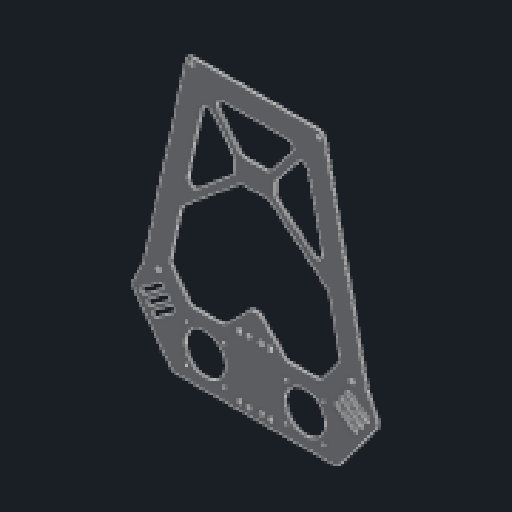
# Autodesk Inventor part: ChestFrontPanel
Saved by Autodesk Inventor 2025.2 (Build 292293000, 293)
## iProperties
Created: 2025-09-23
Part Number: ChestFrontPanel
Material: Generic
Document SubType Name: Sheet Metal
Designer: valer
Density: 1 g/cm^3
Sheet Metal Rule: Default_mm
Appearance: Default
Author: valer
Autodesk Inventor part; units mm, degrees
ref_plane "YZ Plane" through (0, 0, 0) normal (1, 0, 0) x (0, 1, 0)
ref_plane "XZ Plane" through (0, 0, 0) normal (0, 1, 0) x (-1, 0, 0)
ref_plane "XY Plane" through (0, 0, 0) normal (0, 0, 1) x (1, 0, 0)
sketch "Base" plane through (0, 0, 0) normal (0, 0, 1) x (1, 0, 0)
  line L0 (-341.7653, 0) -> (341.7653, 0) construction
  line L1 (0, -75.5138) -> (0, 453.0828) construction
  line L2 (183.676, 264.154) -> (223.6199, 230.6371) construction
  arc A0 (180.154, 267.676) -> (183.676, 264.154) centre (202.0437, 286.0437) ccw construction
  line L3 (105.6111, 356.5128) -> (180.154, 267.676) construction
  arc A1 (105.6111, 356.5128) -> (69.1282, 373.525) centre (69.1282, 325.9) ccw construction
  line L4 (-69.1282, 373.525) -> (69.1282, 373.525) construction
  arc A2 (231.2425, 165.7605) -> (223.6199, 230.6371) centre (193.0071, 194.1542) ccw construction
  line L5 (231.2425, 165.7605) -> (183.8243, 101.9065) construction
  line L6 (0, 373.525) -> (69.1282, 373.525) construction
  line L7 (183.8243, 101.9065) -> (108.1482, 0) construction
  line L8 (108.1482, 0) -> (0, 0) construction
  line L9 (-183.676, 264.154) -> (-223.6199, 230.6371) construction
  arc A3 (-183.676, 264.154) -> (-180.154, 267.676) centre (-202.0437, 286.0437) ccw construction
  line L10 (-105.6111, 356.5128) -> (-180.154, 267.676) construction
  arc A4 (-69.1282, 373.525) -> (-105.6111, 356.5128) centre (-69.1282, 325.9) ccw construction
  arc A5 (-223.6199, 230.6371) -> (-231.2425, 165.7605) centre (-193.0071, 194.1542) ccw construction
  line L11 (-231.2425, 165.7605) -> (-183.8243, 101.9065) construction
  line L12 (0, 373.525) -> (-69.1282, 373.525) construction
  line L13 (-183.8243, 101.9065) -> (-108.1482, 0) construction
  line L14 (-108.1482, 0) -> (0, 0) construction
  circle A6 centre (20.5, 90) radius 3
  line L15 (20.5, 90) -> (8, 90) construction
  line L16 (8, 90) -> (0, 90) construction
  circle A7 centre (8, 90) radius 3
  circle A8 centre (-20.5, 90) radius 3
  line L17 (-20.5, 90) -> (-8, 90) construction
  circle A9 centre (-8, 90) radius 3
  circle A10 centre (90, 16) radius 1.5
  circle A11 centre (90, 65) radius 1.5
  circle A12 centre (41, 16) radius 1.5
  circle A13 centre (41, 65) radius 1.5
  circle A14 centre (65.5, 40.5) radius 25.5 construction
  arc A15 (101, 69) -> (99, 71) centre (99, 69) ccw construction
  line L18 (32, 71) -> (99, 71) construction
  arc A16 (32, 71) -> (30, 69) centre (32, 69) ccw construction
  line L19 (30, 12) -> (30, 69) construction
  arc A17 (30, 12) -> (32, 10) centre (32, 12) ccw construction
  line L20 (99, 10) -> (32, 10) construction
  arc A18 (99, 10) -> (101, 12) centre (99, 12) ccw construction
  line L21 (101, 69) -> (101, 12) construction
  circle A19 centre (-41, 16.5) radius 1.5
  circle A20 centre (-41, 65.5) radius 1.5
  circle A21 centre (-90, 16.5) radius 1.5
  circle A22 centre (-90, 65.5) radius 1.5
  circle A23 centre (-65.5, 41) radius 25.5 construction
  arc A24 (-30, 69.5) -> (-32, 71.5) centre (-32, 69.5) ccw construction
  line L22 (-99, 71.5) -> (-32, 71.5) construction
  arc A25 (-99, 71.5) -> (-101, 69.5) centre (-99, 69.5) ccw construction
  line L23 (-101, 12.5) -> (-101, 69.5) construction
  arc A26 (-101, 12.5) -> (-99, 10.5) centre (-99, 12.5) ccw construction
  line L24 (-32, 10.5) -> (-99, 10.5) construction
  arc A27 (-32, 10.5) -> (-30, 12.5) centre (-32, 12.5) ccw construction
  line L25 (-30, 69.5) -> (-30, 12.5) construction
  line L26 (108.1482, 0) -> (-108.1482, 0)
  line L27 (-108.1482, 0) -> (-186.1215, 105)
  line L28 (-186.1215, 105) -> (186.1215, 105)
  line L29 (186.1215, 105) -> (108.1482, 0)
  circle A28 centre (-65.5, 41) radius 26.5
  circle A29 centre (65.5, 40.5) radius 26.5
  point P0 (0, 0)
  point P1 (0, 105)
  dimension "d6" = 6
  dimension "d7" = 8
  dimension "d8" = 12.5
  dimension "d9" = 90
  dimension "d10" = 15
  dimension "d15" = 1
  dimension "d16" = 1
  measures "d6" diameter of A6
  measures "d7" distance of L15.end L16.end
  measures "d8" distance of L15.start L15.end
  measures "d9" distance between parallel lines of L8 L15
  measures "d10" distance between parallel lines of L28 L15
  measures "d15" radial gap between concentric circles of A28 A23
  measures "d16" radial gap between concentric circles of A29 A14
extrude "Plate1" add sketch "Base" along normal blind 2.54
chamfer "SideChamferFeature" distance 40 angle 45 2 edges at (-186.1215, 105, 1.27) (186.1215, 105, 1.27)
fillet "OutsideFillets1Feature" radius 8 4 edges at (108.1482, 0, 1.27) (162.2738, 72.8863, 1.27) (-108.1482, 0, 1.27) (-162.2738, 72.8863, 1.27)
sketch "Mount" plane through (0, 0, 0) normal (0, 0, -1) x (-1, 0, 0)
  line L0 (-146.1215, 105) -> (146.1215, 105)
  line L1 (-146.1215, 105) -> (-89.2554, 369.0629)
  line L2 (0, -75.5138) -> (0, 453.0828) construction
  line L3 (-89.2554, 369.0629) -> (0, 369.0629)
  arc A0 (-69.1282, 373.525) -> (-105.6111, 356.5128) centre (-69.1282, 325.9) ccw construction
  line L4 (146.1215, 105) -> (89.2554, 369.0629)
  line L5 (89.2554, 369.0629) -> (0, 369.0629)
  point P0 (0, 0)
sheet face with bend "MountFeature" sketch "Mount" thickness 2.54 toward (0, 0, 1) bend radius 2.54 relief straight relief width 2.54 relief depth 1.27
bend "Bend1"
fillet "TopFilletsFeature" radius 8 2 edges at (89.2554, 369.0629, 1.27) (-89.2554, 369.0629, 1.27)
sketch "Cut" plane through (0, 0, 0) normal (0, 0, -1) x (-1, 0, 0)
  line L0 (0, -75.0035) -> (0, 444.6861) construction
  line L1 (-145.9714, 72.7383) -> (-122.689, 90.0279) construction
  line L2 (-143.8847, 69.9284) -> (-120.6023, 87.2179)
  line L3 (-124.7757, 92.8378) -> (-148.0581, 75.5482)
  arc A0 (-148.0581, 75.5482) -> (-143.8847, 69.9284) centre (-145.9714, 72.7383) ccw
  arc A1 (-120.6023, 87.2179) -> (-124.7757, 92.8378) centre (-122.689, 90.0279) ccw
  line L4 (-110.5471, 3.2305) -> (-159.3339, 68.9274) construction
  arc A2 (-113.448, 77.5838) -> (-117.6213, 83.2037) centre (-115.5347, 80.3938) ccw
  line L5 (-117.6213, 83.2037) -> (-140.9037, 65.9141)
  line L6 (-136.7304, 60.2943) -> (-113.448, 77.5838)
  arc A3 (-140.9037, 65.9141) -> (-136.7304, 60.2943) centre (-138.8171, 63.1042) ccw
  arc A4 (-106.2937, 67.9497) -> (-110.467, 73.5696) centre (-108.3804, 70.7597) ccw
  line L7 (-110.467, 73.5696) -> (-133.7494, 56.28)
  line L8 (-129.5761, 50.6602) -> (-106.2937, 67.9497)
  arc A5 (-133.7494, 56.28) -> (-129.5761, 50.6602) centre (-131.6628, 53.4701) ccw
  line L9 (143.8847, 69.9284) -> (120.6023, 87.2179)
  line L10 (124.7757, 92.8378) -> (148.0581, 75.5482)
  arc A6 (143.8847, 69.9284) -> (148.0581, 75.5482) centre (145.9714, 72.7383) ccw
  arc A7 (124.7757, 92.8378) -> (120.6023, 87.2179) centre (122.689, 90.0279) ccw
  arc A8 (117.6213, 83.2037) -> (113.448, 77.5838) centre (115.5347, 80.3938) ccw
  line L11 (117.6213, 83.2037) -> (140.9037, 65.9141)
  line L12 (136.7304, 60.2943) -> (113.448, 77.5838)
  arc A9 (136.7304, 60.2943) -> (140.9037, 65.9141) centre (138.8171, 63.1042) ccw
  arc A10 (110.467, 73.5696) -> (106.2937, 67.9497) centre (108.3804, 70.7597) ccw
  line L13 (110.467, 73.5696) -> (133.7494, 56.28)
  line L14 (129.5761, 50.6602) -> (106.2937, 67.9497)
  arc A11 (129.5761, 50.6602) -> (133.7494, 56.28) centre (131.6628, 53.4701) ccw
  arc A12 (-110.5471, 3.2305) -> (-104.1244, 0) centre (-104.1244, 8) ccw projected
  line L15 (-104.1244, 8) -> (0, 112.1244) construction
  line L16 (104.1244, 0) -> (-104.1244, 0) projected
  line L17 (104.1244, 8) -> (0, 112.1244) construction
  line L18 (-142.5381, 112.1244) -> (142.5381, 112.1244) construction
  line L19 (-160.0581, 77.2916) -> (-146.1215, 105) construction
  line L20 (-65.0282, 339.0629) -> (0, 339.0629)
  line L21 (-65.0282, 339.0629) -> (-111.746, 122.1244)
  line L22 (82.7948, 369.0629) -> (-82.7948, 369.0629) projected
  line L23 (-90.6155, 362.7471) -> (-146.1215, 105) projected
  line L24 (-111.746, 122.1244) -> (0, 122.1244)
  line L25 (65.0282, 339.0629) -> (0, 339.0629)
  line L26 (65.0282, 339.0629) -> (111.746, 122.1244)
  line L27 (111.746, 122.1244) -> (0, 122.1244)
  line L28 (-82.7948, 369.0629) -> (-18.1888, 289.0629)
  line L29 (-90.6155, 362.7471) -> (-26.0096, 282.7471)
  arc A13 (-82.7948, 369.0629) -> (-90.6155, 362.7471) centre (-82.7948, 361.0629) ccw projected
  line L30 (-82.7948, 361.0629) -> (-65.0282, 339.0629) construction
  line L31 (-18.1888, 289.0629) -> (0, 289.0629)
  line L32 (-26.0096, 282.7471) -> (-26.0096, 264.5583)
  line L33 (0, 257.9828) -> (-18.1888, 257.9828)
  line L34 (-26.0096, 282.7471) -> (-18.1888, 289.0629) construction
  line L35 (-26.0096, 264.5583) -> (-18.1888, 257.9828) construction
  line L36 (82.7948, 369.0629) -> (18.1888, 289.0629)
  line L37 (90.6155, 362.7471) -> (26.0096, 282.7471)
  line L38 (18.1888, 289.0629) -> (0, 289.0629)
  line L39 (26.0096, 282.7471) -> (26.0096, 264.5583)
  line L40 (0, 257.9828) -> (18.1888, 257.9828)
  line L41 (-26.0096, 264.5583) -> (-93.0237, 209.0629)
  line L42 (-18.1888, 257.9828) -> (-96.4445, 193.1782)
  line L43 (26.0096, 264.5583) -> (93.0237, 209.0629)
  line L44 (18.1888, 257.9828) -> (96.4445, 193.1782)
  line L45 (-5, 122.1244) -> (-41, 86.1244)
  line L46 (-41, 86.1244) -> (-85.0123, 86.1244)
  line L47 (-85.0123, 86.1244) -> (-111.746, 122.1244)
  line L48 (5, 122.1244) -> (41, 86.1244)
  line L49 (41, 86.1244) -> (85.0123, 86.1244)
  line L50 (85.0123, 86.1244) -> (111.746, 122.1244)
  point P0 (0, 0)
  point P1 (-134.3302, 81.3831)
  point P2 (66.3883, 332.7471)
  point P3 (58.5676, 339.0629)
  point P4 (-58.5676, 339.0629)
  point P5 (-66.3883, 332.7471)
  point P6 (93.0237, 209.0629)
  point P7 (96.4445, 193.1782)
  dimension "d23" = 3.5
  dimension "d24" = 29
  dimension "d25" = 13
  dimension "d26" = 12
  dimension "d29" = 12
  dimension "d34" = 45
  dimension "d35" = 30
  dimension "d36" = 30
  dimension "d37" = 10
  dimension "d38" = 50
  dimension "d39" = 10.0525
  dimension "d50" = 10.0525
  dimension "d51" = 160
  dimension "d52" = 36
  dimension "d53" = 5
  constraints: 92 end point, 31 symmetric about line, 24 point on circle, 12 centre point, 9 point on line, 8 parallel, 7 perpendicular, 4 tangent, 2 equal length, 2 midpoint, 1 horizontal, 27 other
  measures "d23" radius of A1
  measures "d24" distance of L1.start L1.end
  measures "d25" distance from line of L4 L1.start
  measures "d26" horizontal distance of L19.start L3.end
  measures "d29" distance of L1.end A2.centre
  measures "d34" angle of L15 L16
  measures "d35" distance between parallel lines of L23 L21
  measures "d36" distance between parallel lines of L22 L20
  measures "d37" distance between parallel lines of L18 L24
  measures "d38" distance between parallel lines of L20 L31
  measures "d39" distance between parallel lines of L28 L29
  measures "d50" distance between parallel lines of L42 L41
  measures "d51" distance from line of L41.end L22
  measures "d52" distance between parallel lines of L24 L46
  measures "d53" distance from line of L0 L45.start
extrude "CutFeature" cut sketch "Cut" against normal blind 2.54 contours A0 L3 A1 L2 | L6 A3 L5 A2 | L8 A5 L7 A4 | L9 A7 L10 A6 | L11 A9 L12 A8 | L13 A11 L14 A10 | L20 L25 L36 L38 L31 L28 | L29 L32 L41 L21 | L42 L33 L40 L44 L26 L27 L24 L21 | L24 L45 L46 L47 | L26 L43 L39 L37 | L27 L50 L49 L48
fillet "InsideFilletsFeature" radius 8 24 edges at (58.5676, 339.0629, 1.27) (-58.5676, 339.0629, 1.27) (18.1888, 289.0629, 1.27) (-18.1888, 289.0629, 1.27) (66.3883, 332.7471, 1.27) (-66.3883, 332.7471, 1.27) (-26.0096, 282.7471, 1.27) (-26.0096, 264.5583, 1.27) (26.0096, 282.7471, 1.27) (26.0096, 264.5583, 1.27) (18.1888, 257.9828, 1.27) (-18.1888, 257.9828, 1.27) (93.0237, 209.0629, 1.27) (-93.0237, 209.0629, 1.27) (-96.4445, 193.1782, 1.27) (96.4445, 193.1782, 1.27) (111.746, 122.1244, 1.27) (85.0123, 86.1244, 1.27) (41, 86.1244, 1.27) (5, 122.1244, 1.27) (-5, 122.1244, 1.27) (-41, 86.1244, 1.27) (-85.0123, 86.1244, 1.27) (-111.746, 122.1244, 1.27)
sketch "FrameMount" plane through (0, 0, 0) normal (0, 0, -1) x (-1, 0, 0)
  arc A0 (-82.7948, 369.0629) -> (-90.6155, 362.7471) centre (-82.7948, 361.0629) ccw construction
  circle A1 centre (-82.7948, 361.0629) radius 3
  line L0 (-87.8211, 367.2868) -> (-82.7948, 361.0629) construction
  line L1 (0, -74.0889) -> (0, 444.5336) construction
  circle A2 centre (-126.1215, 106.2592) radius 3
  line L2 (-146.1215, 105) -> (-160.0581, 77.2916) construction
  circle A3 centre (82.7948, 361.0629) radius 3
  circle A4 centre (126.1215, 106.2592) radius 3
  line L3 (-87.4112, 89.3549) -> (-109.5849, 119.2143) projected
  point P0 (0, 0)
  dimension "d44" = 6
  dimension "d45" = 8
  dimension "d47" = 6
  dimension "d56" = 20
  dimension "d57" = 21
  constraints: 4 centre point, 2 end point, 2 point on circle, 2 symmetric about line, 1 coincident, 1 point on line, 2 other
  measures "d44" diameter of A1
  measures "d45" distance of A1.centre point (-87.821, 367.287)
  measures "d47" diameter of A2
  measures "d56" horizontal distance of A2.centre L2.start
  measures "d57" distance from line of L3 A2.centre
extrude "FrameMountHolesFeature" cut sketch "FrameMount" against normal blind 2.54
sketch "BottomMountHoles" plane through (0, 0, 0) normal (0, 0, -1) x (-1, 0, 0)
  circle A0 centre (-20.5, 10) radius 3 projected
  circle A1 centre (-8, 10) radius 3 projected
  circle A2 centre (8, 10) radius 3 projected
  circle A3 centre (20.5, 10) radius 3 projected
  point P0 (0, 0)
extrude "BottomMountHolesFeature" cut sketch "BottomMountHoles" against normal blind 2.54
equation "\"d50\" = d39"
equation "\"d41\" = Thickness"
equation "\"d48\" = Thickness"
equation "\"d0\" = Thickness"
equation "\"d17\" = BendRadius"
equation "\"d18\" = BendReliefWidth"
equation "\"d20\" = MinimumRemnant"
equation "\"d19\" = BendReliefDepth"
equation "\"d21\" = TransitionRadius"
equation "\"BendRadius\" = Thickness"
equation "\"BendReliefWidth\" = Thickness"
equation "\"BendReliefDepth\" = 0.5 * Thickness"
equation "\"CornerReliefSize\" = 4 * Thickness"
equation "\"MinimumRemnant\" = 2 * Thickness"
equation "\"TransitionRadius\" = BendRadius"
equation "\"JacobiRadiusSize\" = BendRadius"
equation "\"GapSize\" = Thickness"
equation "\"Thickness\" = 2.54"
body "Solid1"
